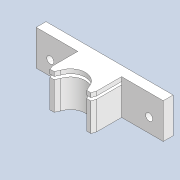
# Autodesk Inventor part: 0008-10-057  Fixare seringa 20 Ml
Saved by Autodesk Inventor 2020 (Build 240168000, 168)
## iProperties
Created: 2021-02-22
Part Number: 0008-10-057  Fixare seringa 20 Ml
Material: ABS Plastic
Document SubType Name: Modeling
Designer: Iulian Bors
Density: 1.06 g/cm^3
Appearance: Smooth - White
Mass: 14.1067 g
Surface Area: 54.8528 cm^2
Volume: 13.3082 cm^3
Description: Fixare Seringa
Author: Iulian Bors
Subject: 004
Autodesk Inventor part; units mm, degrees
ref_plane "YZ Plane" through (0, 0, 0) normal (1, 0, 0) x (0, 1, 0)
ref_plane "XZ Plane" through (0, 0, 0) normal (0, 1, 0) x (-1, 0, 0)
ref_plane "XY Plane" through (0, 0, 0) normal (0, 0, 1) x (1, 0, 0)
sketch "Sketch1" plane through (0, 0, 0) normal (0, 0, 1) x (1, 0, 0)
  line L0 (-45, 10) -> (45, 10)
  line L1 (45, 10) -> (45, -10)
  line L2 (45, -10) -> (-45, -10)
  line L3 (-45, -10) -> (-45, 10)
  point P0 (0, 0)
  point P1 (0, 10)
  point P2 (-45, 0)
  dimension "d0" = 20
  dimension "d1" = 90
  constraints: 8 end point, 2 midpoint, 2 parallel, 1 horizontal, 1 horizontal alignment, 1 perpendicular, 1 vertical alignment
  measures "d0" distance of L2.end L0.start
  measures "d1" distance of L0.start L0.end
extrude "Extrusion1" add sketch "Sketch1" along normal blind 27.75
sketch "Sketch3" plane through (-45, 10, 0) normal (0, 1, 0) x (1, 0, 0)
  line L0 (90, 0) -> (90, -27.75) projected
  line L1 (90, -27.75) -> (0, -27.75) projected
  line L2 (90, -27.75) -> (60.5, -27.75)
  line L3 (60.5, -27.75) -> (60.5, -7)
  line L4 (60.5, -7) -> (90, -7)
  line L5 (90, -7) -> (90, -27.75)
  line L6 (83, -7) -> (95, -7) projected
  line L7 (90, 0) -> (0, 0) projected
  point P0 (45, 0)
  point P1 (60.5, -27.75)
  dimension "d8" = 20.75
  dimension "d20" = 15.5
  dimension "d40" = 7
  constraints: 8 end point, 2 collinear, 2 parallel, 1 horizontal, 1 perpendicular
  measures "d8" distance between parallel lines of L1 L4
  measures "d20" distance from line of L3 point (45, 0)
  measures "d40" distance between parallel lines of L4 L7
extrude "Extrusion2" cut sketch "Sketch3" against normal through all
mirror "Mirror1" about plane through (0, 0, 0) normal (1, 0, 0) of "Extrusion2"
sketch "Sketch4" plane through (-45, 10, 0) normal (0, 1, 0) x (1, 0, 0)
  circle A0 centre (45, -27.75) radius 10.55
  line L0 (90, 0) -> (0, 0) projected
  line L1 (60.5, -27.75) -> (29.5, -27.75) projected
  point P0 (45, 0)
  point P1 (45, 0)
  dimension "d32" = 21.1
  dimension "d39" = 0
  constraints: 2 midpoint, 1 centre point, 1 coincident
  measures "d32" diameter of A0
  measures "d39" distance from line of L1 A0.centre
extrude "Extrusion3" cut sketch "Sketch4" against normal through all
chamfer "Chamfer1" distance 1 distance2 3 1 edges at (-15.5, 0, 27.75) measured on face at (-12.2, -3.3333, 27.75)
chamfer "Chamfer2" distance 1 distance2 3 1 edges at (15.5, 0, 27.75) measured on face at (12.2, 3.3333, 27.75)
sketch "Sketch5" plane through (0, 0, 0) normal (0, 0, -1) x (-1, 0, 0)
  line L0 (45, -10) -> (-45, -10) projected
  line L1 (0, 23.0048) -> (0, -23.0048) construction
  point P0 (0, 0)
  point P1 (-35, 0)
  point P2 (35, 0)
  point P3 (0, 0)
  dimension "d23" = 70
  constraints: 3 horizontal alignment, 2 end point, 1 coincident, 1 midpoint, 1 symmetric about line, 1 vertical
  measures "d23" distance of point (35, 0) point (-35, 0)
hole "Hole1" at (35, 0, 0) at (-35, 0, 0) direction (0, 0, 1) diameter 5 end through all
chamfer "Chamfer3" distance 1 distance2 3 2 edges at (10.55, 0, 27.75) (-10.55, 0, 27.75) measured on face at (13.1833, -3.3333, 27.75) measured on face at (-13.1833, -3.3333, 27.75)
chamfer_without_effect "Chamfer4"
sketch "Sketch6" plane through (-45, 10, 0) normal (0, 1, 0) x (1, 0, 0)
  line L0 (56.55, -27.75) -> (55.1235, -24.7805) projected
  line L1 (59.5, -27.75) -> (56.55, -27.75) projected
  line L2 (60.5, -24.75) -> (59.5, -27.75) projected
  line L3 (60.5, -24.75) -> (60.5, -7) projected
  line L4 (60.5, -7) -> (90, -7) projected
  line L5 (90, 0) -> (90, -7) projected
  line L6 (90, 0) -> (0, 0) projected
  line L7 (0, 0) -> (0, -7) projected
  line L8 (0, -7) -> (29.5, -7) projected
  line L9 (29.5, -7) -> (29.5, -24.75) projected
  line L10 (30.5, -27.75) -> (29.5, -24.75) projected
  line L11 (33.45, -27.75) -> (30.5, -27.75) projected
  line L12 (34.8765, -24.7805) -> (33.45, -27.75) projected
  arc A0 (55.1235, -24.7805) -> (34.8765, -24.7805) centre (45, -27.75) ccw projected
  point P0 (45, 0)
extrude "Extrusion4" add sketch "Sketch6" along normal blind 5
sketch "Sketch7" plane through (-45, -10, 7) normal (0, 0, 1) x (1, 0, 0)
  line L0 (13, 20) -> (27.9, 20) projected
  line L1 (29.5, 22) -> (60.5, 22)
  line L2 (60.5, 22) -> (60.5, 20)
  line L3 (60.5, 20) -> (29.5, 20)
  line L4 (29.5, 20) -> (29.5, 22)
  line L5 (60.5, 25) -> (60.5, 0) projected
  line L6 (29.5, 25) -> (29.5, 0) projected
  point P0 (45, 10)
  dimension "d43" = 2
  constraints: 8 end point, 3 collinear, 2 parallel, 1 horizontal, 1 perpendicular
  measures "d43" distance of L3.end L1.start
extrude "Extrusion5" cut sketch "Sketch7" along normal through all both and the other way through all
body "Solid1"
